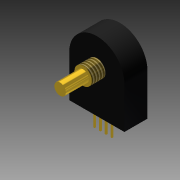
# Autodesk Inventor part: encoder
Saved by Autodesk Inventor 2012 (Build 160160000, 160)
## iProperties
Created: 2012-02-02
Part Number: encoder
Material: Default
Document SubType Name: Modeling
Designer: caduser
Density: 1 g/cm^3
Author: caduser
Autodesk Inventor part; units mm, degrees
ref_plane "YZ Plane" through (0, 0, 0) normal (1, 0, 0) x (0, 1, 0)
ref_plane "XZ Plane" through (0, 0, 0) normal (0, 1, 0) x (-1, 0, 0)
ref_plane "XY Plane" through (0, 0, 0) normal (0, 0, 1) x (1, 0, 0)
sketch "Sketch1" plane through (0, 0, 0) normal (0, 0, 1) x (1, 0, 0)
  line L0 (-21.2649, 0) -> (21.2649, 0) projected
  line L1 (0, -30.5308) -> (0, 22.8092) projected
  arc A0 (15.1892, 0) -> (-15.1892, 0) centre (0, 0) ccw
  line L2 (-15.1892, 0) -> (15.1892, 0)
  line L3 (15.1892, 0) -> (15.1892, -22.9108)
  line L4 (15.1892, -22.9108) -> (-15.1892, -22.9108)
  line L5 (-15.1892, -22.9108) -> (-15.1892, 0)
  dimension "d0" = 30.3784
  dimension "d1" = 38.1
  constraints: 8 end point, 2 parallel, 2 point on circle, 1 centre point, 1 coincident, 1 horizontal, 1 perpendicular, 1 point on line, 1 tangent
  measures "d0" distance of L3.end L4.end
extrude "Extrusion1" add sketch "Sketch1" along normal blind 12.7
sketch "Sketch2" plane through (0, 0, 12.7) normal (0, 0, 1) x (1, 0, 0)
  arc A0 (15.1892, 0) -> (-15.1892, 0) centre (0, 0) ccw projected
  circle A1 centre (0, 0) radius 4.7625
  dimension "d4" = 9.525
  constraints: 1 centre point, 1 coincident
  measures "d4" diameter of A1
extrude "Extrusion2" add sketch "Sketch2" along normal blind 7.5438
sketch "Sketch3" plane through (0, 0, 20.2438) normal (0, 0, 1) x (1, 0, 0)
  circle A0 centre (0, 0) radius 4.7625 projected
  circle A1 centre (0, 0) radius 3.175
  dimension "d7" = 6.35
  constraints: 1 centre point, 1 coincident
  measures "d7" diameter of A1
extrude "Extrusion3" add sketch "Sketch3" along normal blind 12.6492 contours A1
thread "Thread1" size "3/8-16 UNC" class "2A" standard "ANSI Unified Screw Threads" full length
sketch "Sketch4" plane through (-15.1892, -22.9108, 0) normal (0, -1, 0) x (1, 0, 0)
  line L0 (30.3784, 12.7) -> (0, 12.7) projected
  line L1 (0, 0) -> (0, 12.7) projected
  line L2 (10.033, 9.525) -> (10.8267, 9.525)
  line L3 (10.8267, 9.525) -> (10.8267, 8.7313)
  line L4 (10.8267, 8.7313) -> (10.033, 8.7313)
  line L5 (10.033, 8.7313) -> (10.033, 9.525)
  line L6 (13.208, 9.525) -> (14.0017, 9.525)
  line L7 (14.0017, 9.525) -> (14.0017, 8.7313)
  line L8 (14.0017, 8.7313) -> (13.208, 8.7313)
  line L9 (13.208, 8.7313) -> (13.208, 9.525)
  line L10 (16.383, 9.525) -> (17.1767, 9.525)
  line L11 (17.1767, 9.525) -> (17.1767, 8.7313)
  line L12 (17.1767, 8.7313) -> (16.383, 8.7313)
  line L13 (16.383, 8.7313) -> (16.383, 9.525)
  line L14 (19.558, 9.525) -> (20.3517, 9.525)
  line L15 (20.3517, 9.525) -> (20.3517, 8.7313)
  line L16 (20.3517, 8.7313) -> (19.558, 8.7313)
  line L17 (19.558, 8.7313) -> (19.558, 9.525)
  point P0 (15.1892, 0)
  dimension "d12" = 0.7937
  dimension "d13" = 10.033
  dimension "d14" = 3.175
  dimension "d17" = 3.175
  constraints: 32 end point, 2 horizontal, 2 parallel, 2 perpendicular, 24 other
  measures "d12" distance of L2.start L2.end
  measures "d13" distance between parallel lines of L1 L5
  measures "d14" distance between parallel lines of L0 L2
  measures "d17" distance of L3.end L8.start
extrude "Pins" add sketch "Sketch4" along normal blind 9.525
body "Solid1"
